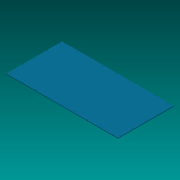
# Autodesk Inventor part: Face A
Saved by Autodesk Inventor 2016 (Build 200138000, 138)
## iProperties
Created: 2015-06-04
Part Number: Face A
Material: ABS Plastic
Document SubType Name: Modeling
Designer: Sawaiz Syed
Density: 1.06 g/cm^3
Appearance: Sky Blue Dark
Author: Sawaiz Syed
Autodesk Inventor part; units mm, degrees
ref_plane "YZ Plane" through (0, 0, 0) normal (1, 0, 0) x (0, 1, 0)
ref_plane "XZ Plane" through (0, 0, 0) normal (0, 1, 0) x (-1, 0, 0)
ref_plane "XY Plane" through (0, 0, 0) normal (0, 0, 1) x (1, 0, 0)
sketch "Sketch1" plane through (0, 0, 0) normal (0, 0, 1) x (1, 0, 0)
  line L0 (-500, -250) -> (500, -250)
  line L1 (500, -250) -> (500, 250)
  line L2 (500, 250) -> (-500, 250)
  line L3 (-500, 250) -> (-500, -250)
  line L4 (-500, -250) -> (500, 250) construction
  line L5 (500, -250) -> (-500, 250) construction
  point P0 (0, 0)
  dimension "d0" = 1000
  dimension "d1" = 500
  constraints: 12 end point, 2 midpoint, 2 parallel, 1 horizontal, 1 perpendicular
  measures "d0" distance of L2.end L1.end
  measures "d1" distance of L1.end L0.end
extrude "Extrusion1" add sketch "Sketch1" along normal blind 4.7625
sketch "Sketch2" plane through (0, 0, 4.7625) normal (0, 0, 1) x (1, 0, 0)
  line L0 (-500, -250) -> (500, -250) projected
  line L1 (500, -250) -> (500, 250) projected
  line L2 (500, 250) -> (-500, 250) projected
  line L3 (-500, 250) -> (-500, -250) projected
  point P0 (0, 0)
  point P1 (-470, 240)
  dimension "d4" = 10
  dimension "d5" = 30
  measures "d4" distance from line of L2 point (-470, 240)
  measures "d5" distance from line of L3 point (-470, 240)
hole "Hole1" at (-470, 240, 4.7625) direction (0, 0, -1) diameter 5 end through all
pattern_linear "Rectangular Pattern1" count 9 spacing 115 along (1, 0, 0) count 2 spacing 480 along (0, -1, 0) of "Hole1"
sketch "Sketch3" plane through (0, 0, 4.7625) normal (0, 0, 1) x (1, 0, 0)
  circle A0 centre (220, -240) radius 2.5 projected
  circle A1 centre (105, -240) radius 2.5 projected
  circle A2 centre (-10, -240) radius 2.5 projected
  circle A3 centre (-125, -240) radius 2.5 projected
  circle A4 centre (-240, -240) radius 2.5 projected
  circle A5 centre (-355, -240) radius 2.5 projected
  circle A6 centre (-470, -240) radius 2.5 projected
  circle A7 centre (220, 240) radius 2.5 projected
  circle A8 centre (105, 240) radius 2.5 projected
  circle A9 centre (-10, 240) radius 2.5 projected
  circle A10 centre (-125, 240) radius 2.5 projected
  circle A11 centre (-240, 240) radius 2.5 projected
  circle A12 centre (-355, 240) radius 2.5 projected
  circle A13 centre (-470, 240) radius 2.5 projected
  line L0 (-500, -250) -> (500, -250) projected
  line L1 (500, -250) -> (500, 250) projected
  line L2 (500, 250) -> (-500, 250) projected
  line L3 (-500, 250) -> (-500, -250) projected
  point P0 (0, 0)
  point P1 (-490, 220)
  dimension "d19" = 10
  dimension "d20" = 30
  measures "d19" distance from line of L3 point (-490, 220)
  measures "d20" distance from line of L2 point (-490, 220)
hole "Hole2" at (-490, 220, 4.7625) direction (0, 0, -1) diameter 5 end through all
pattern_linear "Rectangular Pattern2" count 5 spacing 110 along (0, -1, 0) count 2 spacing 980 along (1, 0, 0) of "Hole2"
body "Solid1"
